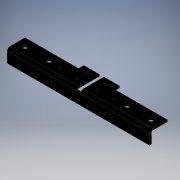
# Autodesk Inventor part: gauge_protection_lateral
Saved by Autodesk Inventor 2018 (Build 220112000, 112)
## iProperties
Created: 2018-06-05
Part Number: gauge_protection_lateral
Material: Generic
Document SubType Name: Sheet Metal
Designer: medrimonia
Density: 1 g/cm^3
Sheet Metal Rule: Default_mm
Sheet Metal Width: 38,000 mm
Sheet Metal Length: 160,000 mm
Sheet Metal Area: 6080,000 mm^2
Appearance: Anodized - Black
Flat Pattern Width: 3.8 cm
Flat Pattern Length: 16 cm
Flat Pattern Area: 60.8 cm^2
Author: medrimonia
Autodesk Inventor part; units mm, degrees
ref_plane "YZ Plane" through (0, 0, 0) normal (1, 0, 0) x (0, 1, 0)
ref_plane "XZ Plane" through (0, 0, 0) normal (0, 1, 0) x (-1, 0, 0)
ref_plane "XY Plane" through (0, 0, 0) normal (0, 0, 1) x (1, 0, 0)
sketch "Sketch2" plane through (0, 0, 0) normal (0, 0, 1) x (1, 0, 0)
  line L0 (-80, 0) -> (80, 0)
  line L1 (80, 0) -> (80, 12)
  line L2 (80, 12) -> (2.5, 12) construction
  line L3 (-80, 12) -> (-80, 0)
  line L4 (80, 12) -> (2.5, 12) construction
  line L5 (2.5, 12) -> (2.5, 32)
  line L6 (2.5, 32) -> (20, 32) construction
  line L7 (80, 32) -> (80, 12)
  line L8 (-2.5, 12) -> (-80, 12) construction
  line L9 (-80, 12) -> (-80, 32)
  line L10 (2.5, 12) -> (-2.5, 12)
  line L11 (-2.5, 12) -> (-80, 12) construction
  line L12 (-2.5, 12) -> (-2.5, 38)
  line L13 (0, 0) -> (0, 12) construction
  line L14 (2.5, 32) -> (2.5, 38)
  line L15 (2.5, 38) -> (20, 38)
  line L16 (20, 38) -> (20, 32)
  line L17 (20, 32) -> (80, 32)
  line L18 (0, 5.9) -> (30, 5.9) construction
  circle A0 centre (30, 5.9) radius 1.5
  circle A1 centre (-30, 5.9) radius 1.5
  line L19 (-80, 12) -> (80, 12)
  line L20 (-80, 32) -> (-20, 32)
  line L21 (-20, 32) -> (-20, 38)
  line L22 (-20, 38) -> (-2.5, 38)
  dimension "d3" = 20
  dimension "d4" = 6
  dimension "d6" = 3
  dimension "d7" = 30
  dimension "d8" = 6.1
  dimension "d10" = 160
  dimension "d11" = 60
  dimension "d12" = 5
  dimension "d42" = 5.9
  constraints: 47 end point, 8 parallel, 7 perpendicular, 6 horizontal, 4 collinear, 2 centre point, 2 midpoint, 2 point on line, 2 vertical, 1 coincident, 1 symmetric about line, 1 other
  measures "d3" distance from line of L7.start L2
  measures "d4" distance of L15.end L6.end
  measures "d6" diameter of A0
  measures "d7" distance of L18.start L18.end
  measures "d8" distance from line of L13.end L18
  measures "d10" distance of L0.start L0.end
  measures "d11" distance of L6.end L7.start
  measures "d12" distance of L12.end L14.end
  measures "d42" distance from line of L0 A1.centre
extrude "Plate2" add sketch "Sketch2" along normal blind 2
fold "Fold2" angle 90 bend radius 1 thickness 2 k factor 0.44 line from (-80, 12, 0) to (80, 12, 0) line at bend end moving side (0, -1, 0) folds toward (0, 0, -1)
sketch "Sketch3" plane through (0, 0, 2) normal (0, 0, 1) x (1, 0, 0)
  line L0 (-80, 14.9531) -> (-2.5, 14.9531) projected
  line L1 (-2.5, 38) -> (-2.5, 14.9531) projected
  line L2 (-20, 38) -> (-2.5, 38) projected
  line L3 (-20, 32) -> (-20, 38) projected
  line L4 (-80, 32) -> (-20, 32) projected
  line L5 (-80, 14.9531) -> (-80, 32) projected
  line L6 (2.5, 14.9531) -> (80, 14.9531) projected
  line L7 (80, 32) -> (80, 14.9531) projected
  line L8 (20, 32) -> (80, 32) projected
  line L9 (20, 38) -> (20, 32) projected
  line L10 (2.5, 38) -> (20, 38) projected
  line L11 (2.5, 14.9531) -> (2.5, 38) projected
  line L12 (80, 11.9531) -> (-80, 11.9531) construction
  line L13 (0, 13.9531) -> (0, 21.9531) construction
  line L14 (0, 21.9531) -> (30, 21.9531) construction
  circle A0 centre (30, 21.9531) radius 1.5
  circle A1 centre (-30, 21.9531) radius 1.5
  line L15 (-2.5, 13.9531) -> (2.5, 13.9531) projected
  point P0 (0, 0)
  dimension "d26" = 3
  dimension "d27" = 30
  dimension "d28" = 8
  constraints: 4 end point, 2 centre point, 1 coincident, 1 midpoint, 1 parallel, 1 perpendicular, 1 symmetric about line, 1 other
  measures "d26" diameter of A0
  measures "d27" distance of L13.end L14.end
  measures "d28" distance of L13.start L13.end
extrude "Extrusion1" cut sketch "Sketch3" against normal through all contours A0 | A1
sketch "Sketch4" plane through (0, 0, 2) normal (0, 0, 1) x (1, 0, 0)
  point P0 (0, 0)
sketch "Sketch5" plane through (0, 0, 2) normal (0, 0, 1) x (1, 0, 0)
  circle A0 centre (30, 21.9531) radius 1.5 projected
  line L0 (2.5, 14.9531) -> (80, 14.9531) projected
  line L1 (80, 32) -> (80, 14.9531) projected
  line L2 (20, 32) -> (80, 32) projected
  line L3 (20, 38) -> (20, 32) projected
  line L4 (2.5, 38) -> (20, 38) projected
  line L5 (2.5, 14.9531) -> (2.5, 38) projected
  circle A1 centre (-30, 21.9531) radius 1.5 projected
  line L6 (-80, 14.9531) -> (-2.5, 14.9531) projected
  line L7 (-2.5, 38) -> (-2.5, 14.9531) projected
  line L8 (-20, 38) -> (-2.5, 38) projected
  line L9 (-20, 32) -> (-20, 38) projected
  line L10 (-80, 32) -> (-20, 32) projected
  line L11 (-80, 14.9531) -> (-80, 32) projected
  line L12 (20, 32) -> (2.5, 32) construction
  circle A2 centre (11.25, 32) radius 1.5
  line L13 (11.25, 32) -> (11.25, 22) construction
  circle A3 centre (11.25, 22) radius 1.5
  line L14 (80, 32) -> (20, 32) construction
  line L15 (80, 14.9531) -> (2.5, 14.9531) construction
  circle A4 centre (43.804, 22.9531) radius 2.5
  circle A5 centre (70.804, 22.9531) radius 2.5
  circle A6 centre (30, 21.9531) radius 1.5 construction
  line L16 (30, 21.9531) -> (43.804, 21.9531) construction
  line L17 (43.804, 21.9531) -> (43.804, 22.9531) construction
  line L18 (43.804, 22.9531) -> (70.804, 22.9531) construction
  dimension "d31" = 3
  dimension "d32" = 10
  dimension "d39" = 13.804
  dimension "d40" = 5
  dimension "d41" = 27
  dimension "d43" = 1
  constraints: 10 end point, 4 centre point, 2 coincident, 2 equal radius, 2 perpendicular, 1 horizontal, 1 midpoint, 1 parallel, 1 point on line, 1 vertical
  measures "d31" diameter of A2
  measures "d32" distance of L13.start L13.end
  measures "d39" distance of L16.start L16.end
  measures "d40" diameter of A4
  measures "d41" distance of L17.end L18.end
  measures "d43" distance between parallel lines of L16 L18
extrude "Extrusion2" cut sketch "Sketch5" against normal through all contours A2 | A3 | A4 | A5
mirror "Mirror1" about plane through (0, 0, 0) normal (1, 0, 0) of "Extrusion2"
equation "\"d13\" = Thickness"
equation "\"d20\" = BendReliefWidth"
equation "\"d21\" = BendReliefDepth"
equation "\"d22\" = MinimumRemnant"
equation "\"d23\" = TransitionRadius"
equation "\"d25\" = bend_radius"
equation "\"d39\" = fixer_2_gauge_hole_x"
equation "\"d41\" = gauge_holes_dist"
equation "\"d43\" = fixer_2_gauge_hole_y"
equation "\"BendRadius\" = Thickness"
equation "\"BendReliefWidth\" = Thickness"
equation "\"BendReliefDepth\" = 0.5 * Thickness"
equation "\"CornerReliefSize\" = 4 * Thickness"
equation "\"MinimumRemnant\" = 2 * Thickness"
equation "\"TransitionRadius\" = BendRadius"
equation "\"JacobiRadiusSize\" = BendRadius"
equation "\"GapSize\" = Thickness"
equation "\"bend_radius\" = 1"
equation "\"fixer_2_gauge_hole_x\" = 13.804"
equation "\"fixer_2_gauge_hole_y\" = 1"
equation "\"gauge_holes_dist\" = 27"
equation "\"Thickness\" = 2"
body "Solid2"
